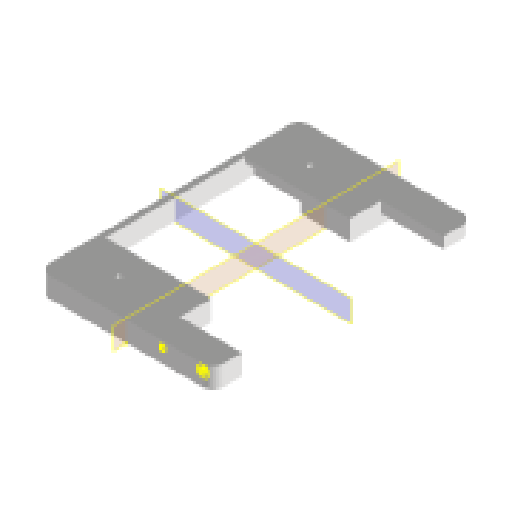
# Autodesk Inventor part: TIRFImager_base_50mm_NEMA11_v3
Saved by Autodesk Inventor 2024.1 (Build 281209000, 209)
## iProperties
Created: 2022-05-21
Part Number: TIRFImager_base_50mm_NEMA11_v3
Material: Generisch
Document SubType Name: Modeling
Designer: diederichbenedict
Density: 1 g/cm^3
Appearance: Vorgabe
Author: diederichbenedict
Autodesk Inventor part; units mm, degrees
ref_plane "YZ Plane" through (0, 0, 0) normal (1, 0, 0) x (0, 1, 0)
ref_plane "XZ Plane" through (0, 0, 0) normal (0, 1, 0) x (-1, 0, 0)
ref_plane "XY Plane" through (0, 0, 0) normal (0, 0, 1) x (1, 0, 0)
sketch "Skizze1" plane through (0, 0, 0) normal (0, 1, 0) x (-1, 0, 0)
  line L0 (-37.75, -63.9) -> (37.75, -63.9)
  line L1 (42.75, -58.9) -> (42.75, 58.9)
  line L2 (37.75, 63.9) -> (-37.75, 63.9)
  line L3 (-42.75, 58.9) -> (-42.75, -58.9)
  line L4 (-42.75, -63.9) -> (42.75, 63.9) construction
  line L5 (42.75, -63.9) -> (-42.75, 63.9) construction
  arc A0 (42.75, 58.9) -> (37.75, 63.9) centre (37.75, 58.9) ccw
  arc A1 (-37.75, 63.9) -> (-42.75, 58.9) centre (-37.75, 58.9) ccw
  arc A2 (-42.75, -58.9) -> (-37.75, -63.9) centre (-37.75, -58.9) ccw
  arc A3 (37.75, -63.9) -> (42.75, -58.9) centre (37.75, -58.9) ccw
  point P0 (0, 0)
  dimension "d0" = 85.5
  dimension "d1" = 127.8
  dimension "d2" = 5
  constraints: 12 end point, 8 point on circle, 8 point on line, 8 tangent, 4 centre point, 3 equal radius, 2 midpoint, 2 parallel, 1 horizontal, 1 perpendicular
  measures "d0" distance of L5.end L4.end
  measures "d1" distance of L4.end L5.start
  measures "d2" radius of A0
extrude "Extrusion1" add sketch "Skizze1" along normal blind 10
ref_plane "Arbeitsebene1" through (37.75, 0, 0) normal (0, 0, -1) x (-1, 0, 0)
ref_plane "Arbeitsebene2" through (0, 0, 58.9) normal (1, 0, 0) x (0, 0, -1)
sketch "Skizze2" plane through (0, 10, 0) normal (0, 1, 0) x (1, 0, 0)
  line L0 (-12.95, 38) -> (-38.75, 38) projected
  line L1 (-38.75, -38) -> (-12.95, -38) projected
  line L2 (-12.95, -38) -> (-12.95, -2.5) projected
  line L3 (-38.75, 38) -> (-38.75, -38) projected
  line L4 (-38.75, -38) -> (-12.95, -38)
  line L5 (-12.95, -38) -> (-12.95, 38)
  line L6 (-12.95, 38) -> (-38.75, 38)
  line L7 (-38.75, 38) -> (-38.75, -38)
  line L8 (-11.95, 39) -> (-11.95, -39)
  line L9 (-11.95, -39) -> (-39.75, -39)
  line L10 (-39.75, -39) -> (-39.75, 39)
  line L11 (-39.75, 39) -> (-11.95, 39)
  line L12 (-11.95, 39) -> (-6.95, 39)
  line L13 (-6.95, 39) -> (-6.95, -39)
  line L14 (-6.95, -39) -> (-11.95, -39)
  line L15 (-11.95, -39) -> (-11.95, 39)
  point P0 (0, 0)
  dimension "d5" = 1
  dimension "d64" = 5
  constraints: 24 end point, 6 parallel, 3 perpendicular, 2 horizontal, 3 other
  measures "d5" distance between parallel lines of L5 L8
  measures "d64" distance between parallel lines of L8 L13
extrude "Extrusion2" cut sketch "Skizze2" against normal through all contours L5 L2 L1 L3 L0 | L12 L13 L14 L8 | L8 L9 L10 L11
ref_plane "Arbeitsebene3" through (-32.75, 5, -38) normal (0, 1, 0) x (0, 0, 1)
sketch "Skizze3" plane through (0, 10, 0) normal (0, 1, 0) x (1, 0, 0)
  line L0 (-39.75, -39) -> (-39.75, 39) projected
  arc A0 (-37.75, 63.9) -> (-42.75, 58.9) centre (-37.75, 58.9) ccw projected
  line L1 (-42.75, 58.9) -> (-42.75, -58.9) projected
  arc A1 (-42.75, -58.9) -> (-37.75, -63.9) centre (-37.75, -58.9) ccw projected
  line L2 (-37.75, -63.9) -> (37.75, -63.9) projected
  arc A2 (37.75, -63.9) -> (42.75, -58.9) centre (37.75, -58.9) ccw projected
  line L3 (42.75, -58.9) -> (42.75, 58.9) projected
  arc A3 (42.75, 58.9) -> (37.75, 63.9) centre (37.75, 58.9) ccw projected
  line L4 (37.75, 63.9) -> (-37.75, 63.9) projected
  line L5 (-39.75, -39) -> (-39.75, 39) projected
  line L6 (-39.75, -39) -> (-6.95, -39)
  line L7 (-6.95, -39) -> (-6.95, -34)
  line L8 (-6.95, -34) -> (-39.75, -34)
  line L9 (-39.75, -34) -> (-39.75, -39)
  line L10 (-39.75, 39) -> (-6.95, 39)
  line L11 (-6.95, 39) -> (-6.95, 34)
  line L12 (-6.95, 34) -> (-39.75, 34)
  line L13 (-39.75, 34) -> (-39.75, 39)
  line L14 (-6.95, -39) -> (-39.75, -39) projected
  line L15 (-39.75, 39) -> (-6.95, 39) projected
  line L16 (-6.95, 39) -> (-6.95, -39) projected
  line L17 (-6.95, -39) -> (-6.95, 39) projected
  point P0 (0, 0)
  dimension "d8" = 32.8
  dimension "d9" = 5
  dimension "d10" = 5
  constraints: 16 end point, 4 parallel, 2 horizontal, 2 perpendicular, 2 point on line
  measures "d8" distance of L8.end L7.end
  measures "d9" distance of L7.end L6.end
  measures "d10" distance of L10.end L11.end
extrude "Extrusion3" add sketch "Skizze3" against normal blind 1 contours L0 L8 L7 L6 | L0 L10 L11 L12
sketch "Skizze4" plane through (0, 0, 0) normal (0, -1, 0) x (1, 0, 0)
  line L0 (-39.75, -39) -> (-39.75, 39) projected
  arc A0 (-42.75, -58.9) -> (-37.75, -63.9) centre (-37.75, -58.9) ccw projected
  line L1 (37.75, -63.9) -> (-37.75, -63.9) projected
  arc A1 (37.75, -63.9) -> (42.75, -58.9) centre (37.75, -58.9) ccw projected
  line L2 (42.75, 58.9) -> (42.75, -58.9) projected
  arc A2 (42.75, 58.9) -> (37.75, 63.9) centre (37.75, 58.9) ccw projected
  line L3 (-37.75, 63.9) -> (37.75, 63.9) projected
  arc A3 (-37.75, 63.9) -> (-42.75, 58.9) centre (-37.75, 58.9) ccw projected
  line L4 (-42.75, -58.9) -> (-42.75, 58.9) projected
  line L5 (-11.95, -34) -> (-11.95, 34) projected
  line L6 (-11.95, 34) -> (12.75, 34)
  line L7 (12.75, 34) -> (12.75, -34)
  line L8 (12.75, -34) -> (-11.95, -34)
  line L9 (-11.95, -34) -> (-11.95, 34)
  line L10 (-2.45, 7.5) -> (-2.45, -8) projected
  line L11 (12.75, -34.1) -> (12.75, -39.1) projected
  line L12 (-39.75, 39) -> (-6.95, 39) projected
  line L13 (-6.95, 39) -> (-6.95, -39) projected
  line L14 (-6.95, -39) -> (-39.75, -39) projected
  point P0 (0, 0)
  dimension "d44" = 0
  constraints: 8 end point, 2 parallel, 1 horizontal, 1 perpendicular, 1 point on line
  measures "d44" distance between parallel lines of L11 L7
extrude "Extrusion4" cut sketch "Skizze4" against normal through all contours L13 L6 L7 L8 | L8 L5 L6 L13
sketch "Skizze5" plane through (0, 0, 0) normal (0, -1, 0) x (1, 0, 0)
  arc A0 (-42.75, -58.9) -> (-37.75, -63.9) centre (-37.75, -58.9) ccw projected
  line L0 (37.75, -63.9) -> (-37.75, -63.9) projected
  arc A1 (37.75, -63.9) -> (42.75, -58.9) centre (37.75, -58.9) ccw projected
  line L1 (42.75, 58.9) -> (42.75, -58.9) projected
  arc A2 (42.75, 58.9) -> (37.75, 63.9) centre (37.75, 58.9) ccw projected
  line L2 (-37.75, 63.9) -> (37.75, 63.9) projected
  arc A3 (-37.75, 63.9) -> (-42.75, 58.9) centre (-37.75, 58.9) ccw projected
  line L3 (-42.75, -58.9) -> (-42.75, 58.9) projected
  line L4 (-6.95, 34) -> (12.75, 34) projected
  line L5 (12.75, 34) -> (12.75, -34) projected
  line L6 (12.75, -34) -> (-6.95, -34) projected
  line L7 (-39.75, -39) -> (-39.75, 39) projected
  circle A4 centre (-19.85, -47) radius 1.4
  circle A5 centre (-19.85, 47) radius 1.4
  line L8 (-6.95, -34) -> (-6.95, -39) projected
  line L9 (-6.95, -39) -> (-39.75, -39) projected
  line L10 (-39.75, 39) -> (-6.95, 39) projected
  line L11 (-6.95, 39) -> (-6.95, 34) projected
  point P0 (0, 0)
  dimension "d18" = 2.8
  dimension "d19" = 2.8
  constraints: 2 centre point
  measures "d18" diameter of A4
  measures "d19" diameter of A5
extrude "Extrusion5" cut sketch "Skizze5" against normal through all contours A4 | A5
sketch "Skizze9" plane through (0, 10, 0) normal (0, -1, 0) x (1, 0, 0)
  circle A0 centre (-19.85, 47) radius 1.4 projected
  circle A1 centre (-19.85, -47) radius 1.4 projected
  arc A2 (-42.75, -58.9) -> (-37.75, -63.9) centre (-37.75, -58.9) ccw projected
  line L0 (37.75, -63.9) -> (-37.75, -63.9) projected
  arc A3 (37.75, -63.9) -> (42.75, -58.9) centre (37.75, -58.9) ccw projected
  line L1 (42.75, 58.9) -> (42.75, -58.9) projected
  arc A4 (42.75, 58.9) -> (37.75, 63.9) centre (37.75, 58.9) ccw projected
  line L2 (-37.75, 63.9) -> (37.75, 63.9) projected
  arc A5 (-37.75, 63.9) -> (-42.75, 58.9) centre (-37.75, 58.9) ccw projected
  line L3 (-42.75, -58.9) -> (-42.75, 58.9) projected
  line L4 (12.75, 34) -> (12.75, -34) projected
  line L5 (12.75, -34) -> (-6.95, -34) projected
  line L6 (-39.75, -39) -> (-39.75, 39) projected
  line L7 (-6.95, 34) -> (12.75, 34) projected
  line L8 (-39.75, 39) -> (-11.95, 39) projected
  line L9 (-39.75, 39) -> (-11.95, 39)
  line L10 (-11.95, 39) -> (-11.95, 34)
  line L11 (-11.95, 34) -> (-39.75, 34)
  line L12 (-39.75, 34) -> (-39.75, 39)
  line L13 (-11.95, -39) -> (-39.75, -39) projected
  line L14 (-39.75, -39) -> (-39.75, -34) projected
  line L15 (-11.95, -39) -> (-39.75, -39)
  line L16 (-39.75, -39) -> (-39.75, -34)
  line L17 (-39.75, -34) -> (-11.95, -34)
  line L18 (-11.95, -34) -> (-11.95, -39)
  line L19 (-39.75, -39) -> (-9.75, -39)
  line L20 (-9.75, -39) -> (-9.75, 39)
  line L21 (-9.75, 39) -> (-39.75, 39)
  line L22 (-39.75, 39) -> (-39.75, -39)
  line L23 (-6.95, -34) -> (-6.95, -39) projected
  line L24 (-6.95, -39) -> (-39.75, -39) projected
  line L25 (-39.75, 39) -> (-6.95, 39) projected
  line L26 (-6.95, 39) -> (-6.95, 34) projected
  point P0 (0, 0)
  dimension "d63" = 30
  constraints: 24 end point, 6 parallel, 3 horizontal, 3 perpendicular
  measures "d63" distance of L21.end L20.end
extrude "Extrusion8" add sketch "Skizze9" along normal blind 1 contours L13 L6 L17 L18
sketch "Skizze10" plane through (0, 10, 0) normal (0, 1, 0) x (1, 0, 0)
  circle A0 centre (36.25, -27.6) radius 1.7 projected
  circle A1 centre (19.25, -27.6) radius 1.7 projected
  circle A2 centre (36.25, 27.4) radius 3.25 projected
  circle A3 centre (19.25, 27.4) radius 3.25 projected
  point P0 (0, 0)
  point P1 (19.25, -37.4)
  point P2 (19.25, 17.6)
  point P3 (36.25, -37.4)
  point P4 (36.25, 17.6)
hole "Bohrung2" at (19.25, 10, 27.6) at (36.25, 10, 27.6) at (19.25, 10, -27.4) at (36.25, 10, -27.4) direction (0, -1, 0) diameter 2.8 end through all
sketch "Skizze11" plane through (42.75, 0, 58.9) normal (1, 0, 0) x (0, 0, -1)
  line L0 (114.8, 0.75) -> (128.8, 0.75) projected
  line L1 (107.8, 0.9) -> (114.8, 0.9) projected
  line L2 (107.8, -26) -> (107.8, 7) projected
  line L3 (9.8, -21) -> (9.8, 7) projected
  line L4 (107.8, 7) -> (9.8, 7)
  line L5 (9.8, 7) -> (9.8, -21)
  line L6 (9.8, -21) -> (107.8, -21)
  line L7 (107.8, -21) -> (107.8, 7)
  line L8 (107.8, 0.9) -> (139.6262, 0.9)
  line L9 (139.6262, 0.9) -> (139.6262, -24.4892)
  line L10 (139.6262, -24.4892) -> (107.8, -24.4892)
  line L11 (107.8, -24.4892) -> (107.8, 0.9)
  line L12 (108.3, -21.5) -> (9.3, -21.5)
  line L13 (9.3, -21.5) -> (9.3, 7.5)
  line L14 (9.3, 7.5) -> (108.3, 7.5)
  line L15 (108.3, 7.5) -> (108.3, -21.5)
  line L16 (107.3, -24.9892) -> (140.1262, -24.9892)
  line L17 (140.1262, -24.9892) -> (140.1262, 1.4)
  line L18 (140.1262, 1.4) -> (107.3, 1.4)
  line L19 (107.3, 1.4) -> (107.3, -24.9892)
  point P0 (58.9, 0)
  point P1 (107.3, -21.5)
  point P2 (108.3, 1.4)
  dimension "d45" = 0.5
  dimension "d46" = 0.5
  constraints: 32 end point, 8 parallel, 4 perpendicular, 2 horizontal, 6 other
  measures "d45" distance between parallel lines of L6 L12
  measures "d46" distance between parallel lines of L10 L16
extrude "Extrusion9" cut sketch "Skizze11" against normal blind 30.5
sketch "Skizze12" plane through (-37.75, 0, 63.9) normal (0, 0, 1) x (1, 0, 0)
  circle A0 centre (75.5, 4) radius 2.75 projected
  circle A1 centre (55.5, 4) radius 1.45 projected
  circle A2 centre (75.5, 4) radius 1.45 projected
  circle A3 centre (55.5, 4) radius 1.45 projected
  point P0 (37.75, 0)
hole "Bohrung3" at (37.75, 4, 63.9) at (17.75, 4, 63.9) direction (0, 0, -1) diameter 3.2 end through all countersink diameter 6 countersink angle 90
sketch "Skizze13" plane through (37.75, 10, -63.9) normal (0, 0, -1) x (-1, 0, 0)
  circle A0 centre (0, -6) radius 2.75 projected
  circle A1 centre (20, -6) radius 2.75 projected
  point P0 (37.75, -10)
hole "Bohrung4" at (37.75, 4, -63.9) at (17.75, 4, -63.9) direction (0, 0, 1) diameter 3.2 end through all countersink diameter 6 countersink angle 90
sketch "Skizze14" plane through (0, 0, 0) normal (0, -1, 0) x (1, 0, 0)
  line L0 (19.35, 62.5) -> (16.15, 62.5) projected
  line L1 (39.35, 62.5) -> (36.15, 62.5) projected
  line L2 (16.15, -62.5) -> (19.35, -62.5) projected
  line L3 (36.15, -62.5) -> (39.35, -62.5) projected
  line L4 (36.2533, -63.9) -> (19.2467, -63.9) projected
  arc A0 (38.9354, -63.7575) -> (42.75, -58.9) centre (37.75, -58.9) ccw projected
  line L5 (42.75, -49.4) -> (42.75, -58.9) projected
  line L6 (42.75, -49.4) -> (12.25, -49.4) projected
  line L7 (12.25, -49.4) -> (12.25, -63.9) projected
  line L8 (16.2533, -63.9) -> (12.25, -63.9) projected
  line L9 (-37.75, 63.9) -> (37.75, 63.9) projected
  line L10 (37.75, -63.9) -> (-37.75, -63.9) projected
  point P0 (0, 0)
  point P1 (17.75, 63.9)
  point P2 (17.75, -63.9)
  constraints: 1 coincident, 1 end point, 1 horizontal alignment, 1 point on line, 1 other
hole "Bohrung5" at (17.75, 0, 63.9) at (37.75, 0, 63.9) at (17.75, 0, -63.9) at (37.75, 0, -63.9) direction (0, 1, 0) diameter 2.8 depth 0.5 tip angle 118
